Self-retaining (two-way) Electromagnet DC 12V Push-pull Solenoid_v3 (Autodesk Fusion 360 design; units mm, degrees)
Autodesk Fusion 360 part; units mm, degrees
sketch "Sketch1" plane through (0, 0, 0) normal (0, 1, 0) x (1, 0, 0)
  line L0 (7.45, -8.575) -> (-7.45, -8.575)
  line L1 (-7.45, -8.575) -> (-7.45, 8.575)
  line L2 (-7.45, 8.575) -> (7.45, 8.575)
  line L3 (7.45, 8.575) -> (7.45, -8.575)
  line L4 (7.45, -8.575) -> (-7.45, 8.575) construction
  line L5 (-7.45, -8.575) -> (7.45, 8.575) construction
  circle A0 centre (0, 0) radius 1
  circle A1 centre (0, 0) radius 1.1
  dimension "d1" = 14.9
  dimension "d2" = 17.15
  dimension "d5" = 2.2
  dimension "d6" = 2
  constraint horizontal L0
  constraint perpendicular L0 L1
  constraint parallel L0 L2
  constraint parallel L1 L3
  constraint coincident L4 A0.centre
  constraint coincident L5 A0.centre
  constraint coincident A0.centre A1.centre
  measures "d1" distance of L1.end L2.end
  measures "d2" distance of L0.end L1.end
  measures "d5" diameter of A1
  measures "d6" diameter of A0
extrude "Extrude1" add sketch "Sketch1" along normal mid plane 22.85 contours L0 L1 L2 L3 makes body 1
extrude "Extrude2" add sketch "Sketch1" along normal blind 42.7 and the other way blind 18.5 from surface at -11.425 separate body contours A0 makes body 2
sketch "Sketch2" plane through (0, -29.925, 0) normal (0, -1, 0) x (1, 0, 0)
  circle A0 centre (0, 0) radius 1
  circle A1 centre (0, 0) radius 2.5
  dimension "d11" = 5
  constraint concentric A0 A1
  measures "d11" diameter of A1
extrude "Extrude3" add sketch "Sketch2" against normal blind 10.78 bodies 1 2
sketch "Sketch3" plane through (0, 31.275, 0) normal (0, 1, 0) x (-1, 0, 0)
  circle A0 centre (0, 0) radius 1
  circle A1 centre (0, 0) radius 2.25
  dimension "d15" = 4.5
  constraint concentric A0 A1
  measures "d15" diameter of A1
extrude "Extrude4" add sketch "Sketch3" against normal blind 14.5 bodies 2
copy_body "Body->Comp1" bodies 1 removing the originals makes body 3 in component "Body"
copy_body "Body->Comp2" bodies 2 removing the originals makes body 4 in component "Rod"
component "Body" placed x (1, 0, 0) y (0, 1, 0) z (0, 0, 1) at (0, 0, 0)
component "Rod" placed x (1, 0, 0) y (0, 1, 0) z (0, 0, 1) at (0, 0, 0)
equation "d5 = d6 + 0.2 mm"
